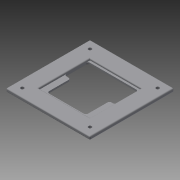
# Autodesk Inventor part: Jig_Power
Saved by Autodesk Inventor 2013 (Build 170138000, 138)
## iProperties
Created: 2013-08-29
Part Number: Jig_Power
Material: Generic
Document SubType Name: Modeling
Designer: md
Density: 1 g/cm^3
Author: md
Autodesk Inventor part; units mm, degrees
ref_plane "YZ Plane" through (0, 0, 0) normal (1, 0, 0) x (0, 1, 0)
ref_plane "XZ Plane" through (0, 0, 0) normal (0, 1, 0) x (-1, 0, 0)
ref_plane "XY Plane" through (0, 0, 0) normal (0, 0, 1) x (1, 0, 0)
sketch "Sketch1" plane through (0, 0, 0) normal (0, 0, 1) x (1, 0, 0)
  line L0 (-25, 25) -> (25, 25)
  line L1 (25, 25) -> (25, -25)
  line L2 (25, -25) -> (-25, -25)
  line L3 (-25, -25) -> (-25, 25)
  line L4 (-25, 25) -> (25, -25) construction
  line L5 (25, 25) -> (-25, -25) construction
  line L6 (-41, 41) -> (41, 41)
  line L7 (41, 41) -> (41, -41)
  line L8 (41, -41) -> (-41, -41)
  line L9 (-41, -41) -> (-41, 41)
  line L10 (-41, 41) -> (41, -41) construction
  line L11 (41, 41) -> (-41, -41) construction
  line L12 (-33, -33) -> (33, -33) construction
  line L13 (33, -33) -> (33, 33) construction
  line L14 (33, 33) -> (-33, 33) construction
  line L15 (-33, 33) -> (-33, -33) construction
  line L16 (-33, -33) -> (33, 33) construction
  line L17 (33, -33) -> (-33, 33) construction
  circle A0 centre (-33, 33) radius 1.6
  circle A1 centre (33, 33) radius 1.6
  circle A2 centre (33, -33) radius 1.6
  circle A3 centre (-33, -33) radius 1.6
  point P0 (0, 0)
  dimension "d0" = 50
  dimension "d1" = 50
  dimension "d2" = 16
  dimension "d3" = 8
  dimension "d4" = 16
  dimension "d5" = 3.2
  constraints: 36 end point, 6 midpoint, 6 parallel, 4 centre point, 4 coincident, 3 equal radius, 3 horizontal, 3 perpendicular, 1 point on line
  measures "d0" distance of L1.end L2.end
  measures "d1" distance of L0.end L1.end
  measures "d2" distance between parallel lines of L6 L0
  measures "d3" distance between parallel lines of L6 L14
  measures "d4" distance between parallel lines of L1 L7
  measures "d5" diameter of A0
extrude "Extrusion1" add sketch "Sketch1" along normal blind 1.7
sketch "Sketch2" plane through (0, 0, 0) normal (0, 0, -1) x (-1, 0, 0)
  line L0 (-25, -25) -> (-25, 25) projected
  line L1 (-25, 25) -> (25, 25) projected
  line L2 (25, 25) -> (25, -25) projected
  line L3 (25, -25) -> (-25, -25) projected
  circle A0 centre (33, -33) radius 1.6 projected
  circle A1 centre (-33, -33) radius 1.6 projected
  circle A2 centre (-33, 33) radius 1.6 projected
  circle A3 centre (33, 33) radius 1.6 projected
  line L4 (41, 41) -> (-41, 41) projected
  line L5 (-41, 41) -> (-41, -41) projected
  line L6 (-41, -41) -> (41, -41) projected
  line L7 (41, -41) -> (41, 41) projected
  line L8 (-24.2, 21) -> (-24.2, 2)
  line L9 (-17, -23) -> (17, -23)
  line L10 (19, -21) -> (19, -2)
  line L11 (23, 23) -> (-22.2, 23)
  line L12 (21, 0) -> (23, 0)
  line L13 (-22.2, 0) -> (-21, 0)
  line L14 (-19, -2) -> (-19, -21)
  arc A4 (-22.2, 23) -> (-24.2, 21) centre (-22.2, 21) ccw
  arc A5 (-24.2, 2) -> (-22.2, 0) centre (-22.2, 2) ccw
  arc A6 (-19, -2) -> (-21, 0) centre (-21, -2) ccw
  arc A7 (-19, -21) -> (-17, -23) centre (-17, -21) ccw
  arc A8 (17, -23) -> (19, -21) centre (17, -21) ccw
  arc A9 (21, 0) -> (19, -2) centre (21, -2) ccw
  line L15 (25, 21) -> (25, 2)
  arc A10 (25, 21) -> (23, 23) centre (23, 21) ccw
  arc A11 (23, 0) -> (25, 2) centre (23, 2) ccw
  point P0 (0, 0)
  point P1 (25, 23)
  point P2 (25, 0)
  dimension "d8" = 0.8
  dimension "d9" = 6
  dimension "d10" = 6
  dimension "d11" = 2
  dimension "d12" = 2
  dimension "d13" = 41
  dimension "d14" = 2
  dimension "d15" = 2
  constraints: 16 end point, 16 point on circle, 16 tangent, 8 centre point, 6 equal radius, 5 point on line, 2 collinear, 2 perpendicular, 1 midpoint
  measures "d8" distance between parallel lines of L0 L8
  measures "d9" distance between parallel lines of L0 L14
  measures "d10" distance between parallel lines of L2 L10
  measures "d11" distance between parallel lines of L3 L9
  measures "d12" distance between parallel lines of L1 L11
  measures "d13" distance between parallel lines of L4 L13
  measures "d14" radius of A4
  measures "d15" radius of A10
extrude "Extrusion2" add sketch "Sketch2" along normal blind 1.7 contours L0 L1 L2 A10 L11 A4 L8 A5 L13 A6 L14 A7 L9 A8 L10 A9 L12 A11 L3 | L7 L6 L5 L4
fillet "Fillet1" radius 1 12 edges at (0, 41, 1.7) (-41, 0, 1.7) (0, -41, 1.7) (41, 0, 1.7) (0, 41, -1.7) (41, 0, -1.7) (0, -41, -1.7) (-41, 0, -1.7) (25, 0, 1.7) (0, -25, 1.7) (-25, 0, 1.7) (0, 25, 1.7)
fillet "Fillet2" radius 1 12 edges at (-40.7071, -40.7071, -1.4071) (-40.7071, -40.7071, 1.4071) (-41, -41, 0) (41, -41, 0) (40.7071, -40.7071, -1.4071) (40.7071, -40.7071, 1.4071) (41, 41, 0) (40.7071, 40.7071, -1.4071) (40.7071, 40.7071, 1.4071) (-40.7071, 40.7071, 1.4071) (-40.7071, 40.7071, -1.4071) (-41, 41, 0)
equation "\"d3\" = 0.5 * d2"
equation "\"d4\" = d2"
equation "\"d10\" = d9"
equation "\"d11\" = d12"
body "Solid1"
